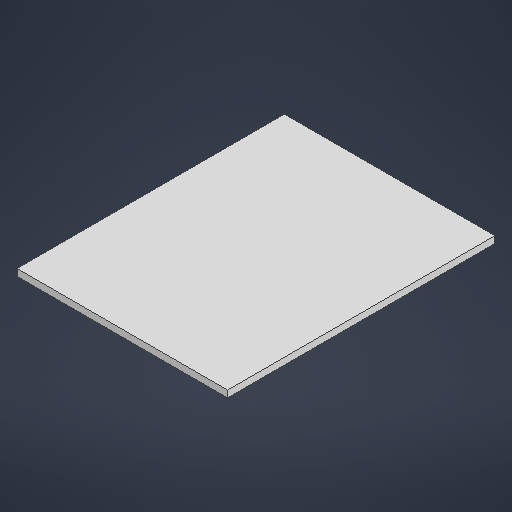
# Autodesk Inventor part: Shelf
Saved by Autodesk Inventor 2026.2 (Build 302298010, 298A)
## iProperties
Created: 2026-08-24
Part Number: Shelf
Material: Generic
Document SubType Name: Modeling
Designer: aiden
Density: 1 g/cm^3
Appearance: Default
Author: aiden
Autodesk Inventor part; units mm, degrees
ref_plane "YZ Plane" through (0, 0, 0) normal (1, 0, 0) x (0, 1, 0)
ref_plane "XZ Plane" through (0, 0, 0) normal (0, 1, 0) x (-1, 0, 0)
ref_plane "XY Plane" through (0, 0, 0) normal (0, 0, 1) x (1, 0, 0)
sketch "Sketch1" plane through (0, 0, 0) normal (0, 1, 0) x (-1, 0, 0)
  line L0 (-155, -196.85) -> (155, -196.85)
  line L1 (155, -196.85) -> (155, 196.85)
  line L2 (155, 196.85) -> (-155, 196.85)
  line L3 (-155, 196.85) -> (-155, -196.85)
  line L4 (-155, -196.85) -> (155, 196.85) construction
  line L5 (155, -196.85) -> (-155, 196.85) construction
  point P0 (0, 0)
  dimension "d0" = 310
  dimension "d1" = 393.7
  constraints: 12 end point, 2 midpoint, 2 parallel, 1 horizontal, 1 perpendicular
  measures "d0" distance of L2.end L1.end
  measures "d1" distance of L1.end L0.end
extrude "Extrusion1" add sketch "Sketch1" along normal blind 10
body "Solid1"
